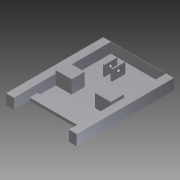
# Autodesk Inventor part: Concept
Saved by Autodesk Inventor 2012 (Build 160160000, 160)
## iProperties
Created: 2011-09-11
Part Number: Concept
Material: Default
Document SubType Name: Modeling
Designer: Ian Walters
Density: 1 g/cm^3
Author: Ian Walters
Autodesk Inventor part; units mm, degrees
ref_plane "YZ Plane" through (0, 0, 0) normal (1, 0, 0) x (0, 1, 0)
ref_plane "XZ Plane" through (0, 0, 0) normal (0, 1, 0) x (-1, 0, 0)
ref_plane "XY Plane" through (0, 0, 0) normal (0, 0, 1) x (1, 0, 0)
sketch "Sketch1" plane through (0, 0, 0) normal (0, 0, 1) x (1, 0, 0)
  line L0 (-266.7, 101.6) -> (-342.9, 101.6)
  line L1 (-342.9, 101.6) -> (-342.9, 0)
  line L2 (-342.9, 0) -> (342.9, 0)
  line L3 (342.9, 0) -> (342.9, 101.6)
  line L4 (342.9, 101.6) -> (266.7, 101.6)
  line L5 (266.7, 101.6) -> (266.7, 2.54)
  line L6 (266.7, 2.54) -> (-266.7, 2.54)
  line L7 (-266.7, 2.54) -> (-266.7, 101.6)
  point P0 (0, 0)
  point P1 (0, 0)
  point P2 (0, 2.54)
  dimension "d0" = 685.8
  dimension "d1" = 101.6
  dimension "d2" = 76.2
  dimension "d3" = 2.54
  constraints: 16 end point, 5 parallel, 2 collinear, 2 midpoint, 1 coincident, 1 horizontal, 1 perpendicular, 1 vertical alignment
  measures "d0" distance of L1.end L2.end
  measures "d1" distance of L0.end L1.end
  measures "d2" distance of L0.start L0.end
  measures "d3" distance between parallel lines of L2 L6
extrude "Extrusion1" add sketch "Sketch1" along normal mid plane 939.8
sketch "Sketch2" plane through (0, 0, -469.9) normal (0, 0, -1) x (-1, 0, 0)
  line L0 (-342.9, 0) -> (-342.9, 101.6) projected
  line L1 (342.9, 0) -> (-342.9, 0) projected
  line L2 (-342.9, 101.6) -> (342.9, 101.6)
  line L3 (342.9, 101.6) -> (342.9, 0)
  line L4 (342.9, 0) -> (-342.9, 0)
  line L5 (-342.9, 0) -> (-342.9, 101.6)
  point P0 (0, 0)
  constraints: 8 end point, 2 parallel, 1 horizontal, 1 perpendicular
extrude "Extrusion2" add sketch "Sketch2" along normal blind 2.54
sketch "Sketch3" plane through (-266.7, 2.54, 469.9) normal (0, 1, 0) x (1, 0, 0)
  line L0 (0, 0) -> (533.4, 0) projected
  line L1 (533.4, 939.8) -> (533.4, 0) projected
  line L2 (0, 939.8) -> (0, 0) projected
  line L3 (0, 152.4) -> (533.4, 152.4)
  line L4 (533.4, 152.4) -> (533.4, 228.6)
  line L5 (533.4, 228.6) -> (0, 228.6)
  line L6 (0, 228.6) -> (0, 152.4)
  line L7 (0, 533.4) -> (152.4, 533.4)
  line L8 (152.4, 533.4) -> (152.4, 406.4)
  line L9 (152.4, 406.4) -> (0, 406.4)
  line L10 (0, 406.4) -> (0, 533.4)
  line L11 (381, 533.4) -> (533.4, 533.4)
  line L12 (533.4, 533.4) -> (533.4, 406.4)
  line L13 (533.4, 406.4) -> (381, 406.4)
  line L14 (381, 406.4) -> (381, 533.4)
  point P0 (266.7, 469.9)
  point P1 (152.4, 469.9)
  dimension "d8" = 76.2
  dimension "d9" = 152.4
  dimension "d31" = 152.4
  dimension "d32" = 127
  constraints: 24 end point, 6 parallel, 5 point on line, 3 horizontal, 3 perpendicular, 2 equal length, 1 collinear, 1 horizontal alignment, 1 midpoint
  measures "d8" distance of L5.end L3.start
  measures "d9" distance between parallel lines of L0 L3
  measures "d31" distance of L8.end L9.end
  measures "d32" distance of L7.end L8.end
extrude "Extrusion7" cut sketch "Sketch3" against normal up to next contours L2 L3 L1 L0
extrude "Extrusion3" add sketch "Sketch3" along normal blind 25.4 contours L2 L5 L1 L3
extrude "Extrusion8" add sketch "Sketch3" along normal blind 127 contours L1 L13 L14 L11 | L7 L8 L9 L2
sketch "Sketch4" plane through (-342.9, 0, 469.9) normal (0, -1, 0) x (1, 0, 0)
  line L0 (685.8, 0) -> (0, 0) projected
  line L1 (0, -942.34) -> (0, 0) projected
  line L2 (0, -942.34) -> (685.8, -942.34) projected
  line L3 (76.2, -939.8) -> (76.2, -228.6) projected
  line L4 (342.9, -469.9) -> (342.9, 0) construction
  line L5 (12.7, -929.64) -> (63.5, -929.64)
  line L6 (63.5, -929.64) -> (63.5, -12.7)
  line L7 (63.5, -12.7) -> (12.7, -12.7)
  line L8 (12.7, -12.7) -> (12.7, -929.64)
  line L9 (673.1, -929.64) -> (622.3, -929.64)
  line L10 (622.3, -929.64) -> (622.3, -12.7)
  line L11 (622.3, -12.7) -> (673.1, -12.7)
  line L12 (673.1, -12.7) -> (673.1, -929.64)
  dimension "d12" = 12.7
  dimension "d13" = 12.7
  dimension "d14" = 12.7
  dimension "d15" = 12.7
  constraints: 18 end point, 4 symmetric about line, 2 parallel, 1 horizontal, 1 midpoint, 1 perpendicular
  measures "d12" distance between parallel lines of L1 L8
  measures "d13" distance between parallel lines of L3 L6
  measures "d14" distance between parallel lines of L0 L7
  measures "d15" distance between parallel lines of L5 L2
extrude "Extrusion4" cut sketch "Sketch4" against normal blind 88.9
sketch "Sketch5" plane through (-266.7, 2.54, -469.9) normal (0, 1, 0) x (1, 0, 0)
  line L0 (533.4, 0) -> (0, 0) projected
  line L1 (0, 0) -> (0, -711.2) projected
  line L2 (152.4, -101.6) -> (165.1, -101.6)
  line L3 (165.1, -101.6) -> (165.1, -228.6)
  line L4 (165.1, -228.6) -> (152.4, -228.6)
  line L5 (152.4, -228.6) -> (152.4, -101.6)
  line L6 (228.6, -101.6) -> (241.3, -101.6)
  line L7 (241.3, -101.6) -> (241.3, -228.6)
  line L8 (241.3, -228.6) -> (228.6, -228.6)
  line L9 (228.6, -228.6) -> (228.6, -101.6)
  point P0 (266.7, -469.9)
  dimension "d18" = 12.7
  dimension "d19" = 127
  dimension "d20" = 63.5
  dimension "d21" = 152.4
  dimension "d22" = 101.6
  constraints: 16 end point, 4 parallel, 2 equal length, 2 horizontal, 2 perpendicular, 1 horizontal alignment
  measures "d18" distance of L3.end L4.end
  measures "d19" distance of L2.end L3.end
  measures "d20" distance between parallel lines of L9 L3
  measures "d21" distance between parallel lines of L1 L5
  measures "d22" distance between parallel lines of L0 L2
extrude "Extrusion5" add sketch "Sketch5" along normal blind 101.6
sketch "Sketch6" plane through (-25.4, 2.54, -241.3) normal (1, 0, 0) x (0, 0, -1)
  line L0 (127, 101.6) -> (0, 101.6) projected
  circle A0 centre (63.5, 63.5) radius 14.2875
  point P0 (-241.3, -2.54)
  point P1 (63.5, 101.6)
  dimension "d25" = 28.575
  dimension "d26" = 38.1
  constraints: 1 centre point, 1 midpoint, 1 vertical alignment
  measures "d25" diameter of A0
  measures "d26" distance from line of L0 A0.centre
extrude "Extrusion6" cut sketch "Sketch6" against normal up to surface (88.9 mm away)
body "Solid1"
